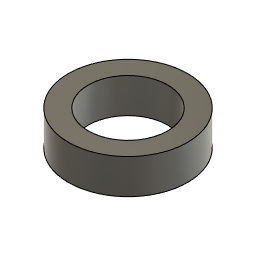
Motor and spindle gear (Autodesk Fusion 360 archive; units mm, degrees)
design "MR128ZZ Ball Bearing"
Autodesk Fusion 360 part; units mm, degrees
sketch "Sketch1" plane through (0, 0, 0) normal (0, 1, 0) x (1, 0, 0)
  circle A0 centre (0, 0) radius 4
  circle A1 centre (0, 0) radius 6
  dimension "d1" = 8
  dimension "d2" = 12
  constraint coincident A0.centre A1.centre
  measures "d1" diameter of A0
  measures "d2" diameter of A1
extrude "Extrude1" add sketch "Sketch1" along normal blind 3.5

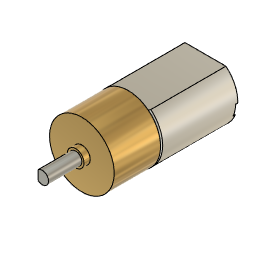
design "GA16-030 Gear Motor"
Autodesk Fusion 360 part; units mm, degrees
sketch "Sketch1" plane through (0, 0, 0) normal (0, 1, 0) x (1, 0, 0)
  circle A0 centre (0, 0) radius 7.75
  circle A1 centre (0, 0) radius 2
  circle A2 centre (0, 0) radius 1.5
  line L0 (-1, -1.118) -> (-1, 1.118)
  line L1 (-4.9054, -6) -> (4.9054, -6)
  line L2 (4.9054, -6) -> (4.9054, 6) construction
  line L3 (4.9054, 6) -> (-4.9054, 6)
  line L4 (-4.9054, 6) -> (-4.9054, -6) construction
  dimension "d1" = 15.5
  dimension "d2" = 4
  dimension "d3" = 3
  dimension "d4" = 2.5
  dimension "d5" = 12
  constraint coincident A0.centre A1.centre
  constraint concentric A1 A2
  constraint coincident A2 L0.start
  constraint coincident A2 L0.end
  constraint vertical L0
  constraint horizontal L1
  constraint vertical L2
  constraint horizontal L3
  constraint vertical L4
  constraint coincident A0 L2.end
  constraint coincident A0 L1.start
  constraint coincident A0 L1.end
  measures "d1" diameter of A0
  measures "d2" diameter of A1
  measures "d3" diameter of A2
  measures "d5" distance of L1.end L2.end
extrude "Extrude1" add sketch "Sketch1" along normal blind 11.1 contours A0 L1 L3 | A0 L3 | A0 L1 | A1 | A2 L0 | A2 L0 makes body 1
extrude "Extrude2" add sketch "Sketch1" along normal blind 18.5 from surface at 11.1 separate body contours A0 L1 L3 | A1 | A2 L0 | A2 L0 makes body 2
fillet "Fillet1" radius 0.5 2 edges at (7.75, 11.1, 0) (-7.75, 11.1, 0) on bodies 2
extrude "Extrude4" add sketch "Sketch1" against normal blind 1.5 contours A1 bodies 1
extrude "Extrude3" add sketch "Sketch1" against normal blind 9.5 separate body contours A2 L0 picked at (-0.2904, 0.3293) makes body 3
extrude "Extrude8" add sketch "Sketch1" against normal blind 3 contours A2 L0 picked at (-1.1959, 0.1886) bodies 3
sketch "Sketch2" plane through (0, 29.6, 0) normal (0, 1, 0) x (-1, 0, 0)
  circle A0 centre (0, 0) radius 2.75
  line L0 (3.9347, 0.9533) -> (4.3966, 1.1447)
  line L1 (4.3966, 1.1447) -> (4.9707, -0.2412)
  line L2 (4.9707, -0.2412) -> (4.5087, -0.4325)
  line L3 (4.5087, -0.4325) -> (3.9347, 0.9533)
  line L4 (1.0524, -2.5407) -> (7.7465, 0.2321)
  line L5 (-7.1601, -2.9658) -> (7.1601, 2.9658)
  line L6 (0, 0) -> (7.75, 0) construction
  line L7 (0.5262, -1.2703) -> (4.6836, 0.4517) construction
  line L8 (0, 0) -> (1.0524, -2.5407) construction
  line L9 (-4.5087, 0.4325) -> (-3.9347, -0.9533)
  line L10 (-3.9347, -0.9533) -> (-4.3966, -1.1447)
  line L11 (-4.3966, -1.1447) -> (-4.9707, 0.2412)
  line L12 (-4.9707, 0.2412) -> (-4.5087, 0.4325)
  line L13 (-1.0524, 2.5407) -> (-7.7465, -0.2321)
  arc A1 (-4.9054, 6) -> (-4.9054, -6) centre (0, 0) ccw
  line L14 (-4.9054, -6) -> (4.9054, -6)
  arc A2 (4.9054, -6) -> (4.9054, 6) centre (0, 0) ccw
  line L15 (4.9054, 6) -> (-4.9054, 6)
  dimension "d17" = 5.5
  dimension "d26" = 22.5
  dimension "d27" = 1.5
  dimension "d28" = 0.5
  dimension "d29" = 4.5
  dimension "d31" = 360
  dimension "d37" = 9
  dimension "d38" = 4.25
  constraint coincident A0 L4.start
  constraint midpoint A0.centre L5
  constraint parallel L4 L5
  constraint tangent A0 L4
  constraint coincident A0.centre L6.start
  constraint parallel L5 L7
  constraint perpendicular L0 L3
  constraint perpendicular L0 L1
  constraint perpendicular L3 L7
  constraint perpendicular L2 L3
  constraint midpoint L7.start L8
  constraint midpoint L1 L7.end
  constraint coincident L5.end A2
  constraint horizontal L6
  constraint coincident L4.end A2
  constraint midpoint L6.end A2
  measures "d17" diameter of A0
  measures "d26" angle of L5 L6
  measures "d27" distance of L0.end L1.end
  measures "d28" distance of L1.end L2.end
  measures "d29" distance of L7.start L7.end
  measures "d37" distance of L1 L11
  measures "d38" distance of L2 L12
extrude "Extrude7" cut sketch "Sketch2" against normal blind 0.5 contours A0 L4 L5 A2 | A0 L5 L13 A1 | L0 L1 L2 L3 | L9 L10 L11 L12 bodies 2
extrude "Extrude5" add sketch "Sketch2" along normal blind 2 and the other way up to surface (0.5 mm away) separate body contours L0 L1 L2 L3 | L9 L10 L11 L12 makes body 4 at (-4.126, 30.7667, 0.4914) makes body 5 at (4.588, 29.9333, -0.6827)
extrude "Extrude6" add sketch "Sketch2" along normal blind 1 contours A0 L5 | A0 L5 bodies 2 1
